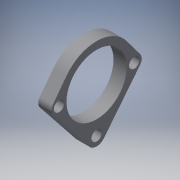
# Autodesk Inventor part: F6804 Holder
Saved by Autodesk Inventor 2019.4 (Build 234330000, 330)
## iProperties
Created: 2019-12-12
Part Number: F6804 Holder
Material: Aluminum 6061
Document SubType Name: Modeling
Designer: Mark
Mass: 10.8578 g
Surface Area: 32.1156 cm^2
Volume: 4.02142 cm^3
Density: 2.7 g/cm^3
Appearance: Aluminum - Flat
Author: Mark
Autodesk Inventor part; units mm, degrees
ref_plane "YZ Plane" through (0, 0, 0) normal (1, 0, 0) x (0, 1, 0)
ref_plane "XZ Plane" through (0, 0, 0) normal (0, 1, 0) x (-1, 0, 0)
ref_plane "XY Plane" through (0, 0, 0) normal (0, 0, 1) x (1, 0, 0)
sketch "Sketch1" plane through (0, 0, 0) normal (1, 0, 0) x (0, 1, 0)
  circle A0 centre (0, 0) radius 16
  line L0 (0, 0) -> (-20, 0) construction
  line L1 (0, 0) -> (20, 0) construction
  circle A1 centre (-23.5, 0) radius 3.5 construction
  circle A2 centre (-23.5, 0) radius 2.75
  arc A3 (-26.6155, 3.9107) -> (-26.6155, -3.9107) centre (-23.5, 0) ccw
  line L2 (-26.6155, -3.9107) -> (-12.2395, -15.3635)
  line L3 (-26.6155, 3.9107) -> (-12.2395, 15.3635)
  circle A4 centre (0, -20) radius 2.75
  arc A5 (-2.4924, -23.1286) -> (2.4, -23.2) centre (0, -20) ccw
  line L4 (0, 0) -> (0, -30) construction
  line L5 (2.4, -23.2) -> (12, -16)
  line L6 (-2.4924, -23.1286) -> (-12.2395, -15.3635)
  line L7 (2.4, 23.2) -> (12, 16)
  circle A6 centre (0, 20) radius 2.75
  arc A7 (2.4, 23.2) -> (-2.4924, 23.1286) centre (0, 20) ccw
  line L8 (-2.4924, 23.1286) -> (-12.2395, 15.3635)
  arc A8 (-12.2395, -15.3635) -> (-12.2395, -15.3635) centre (0, 0) ccw
  arc A9 (-12.2395, 15.3635) -> (-12.2395, 15.3635) centre (0, 0) ccw
  arc A10 (12, -16) -> (12, 16) centre (0, 0) ccw
  dimension "d4" = 7
  dimension "d1" = 32
  dimension "d3" = 180
  dimension "d5" = 5.5
  dimension "d6" = 10
  dimension "d8" = 5.5
  dimension "d9" = 30
  dimension "d10" = 23.5
  dimension "d11" = 20
  dimension "d12" = 20
  constraints: 18 end point, 12 point on circle, 10 centre point, 8 symmetric about line, 7 coincident, 7 tangent, 2 collinear, 2 horizontal, 2 point on line, 1 horizontal alignment, 1 vertical, 4 other
  measures "d1" diameter of A0
  measures "d3" angle of L0 L1
  measures "d5" diameter of A2
  measures "d6" diameter of A3
  measures "d8" diameter of A4
  measures "d9" distance of L4.start L4.end
  measures "d10" distance of point (0, 0) point (-23.5, 0)
  measures "d11" distance of point (0, 0) A4.centre
  measures "d12" radius of A10
extrude "Extrusion1" add sketch "Sketch1" along normal blind 7 contours L3 A8 L2 A3 | A8 A6 A4 | L8 A7 L7 A10 L5 A5 L6 A8 A4 A6
body "Solid1"
